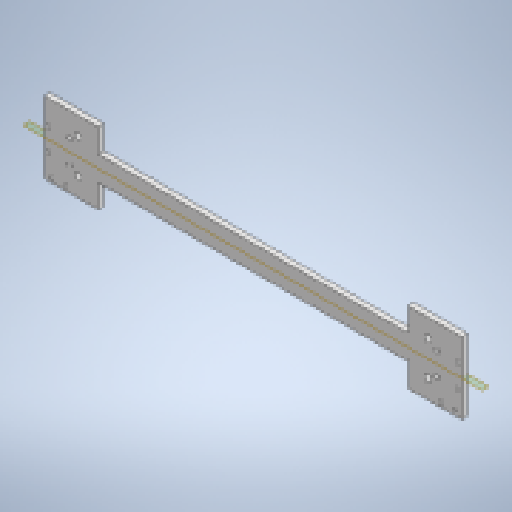
# Autodesk Inventor part: центр_рейка
Saved by Autodesk Inventor 2023.1 (Build 271208000, 208)
## iProperties
Created: 2025-12-22
Part Number: центр_рейка
Material: Типовые
Document SubType Name: Modeling
Designer: DELL
Density: 1 g/cm^3
Appearance: По умолчанию
Author: DELL
Autodesk Inventor part; units mm, degrees
ref_plane "YZ Plane" through (0, 0, 0) normal (1, 0, 0) x (0, 1, 0)
ref_plane "XZ Plane" through (0, 0, 0) normal (0, 1, 0) x (-1, 0, 0)
ref_plane "XY Plane" through (0, 0, 0) normal (0, 0, 1) x (1, 0, 0)
sketch "Эскиз1" plane through (0, 0, 0) normal (0, 0, 1) x (1, 0, 0)
  circle A0 centre (-7.5, -22.95) radius 1.5 projected
  circle A1 centre (7.5, -22.95) radius 1.5 projected
  circle A2 centre (7.5, -6.95) radius 1.5 projected
  circle A3 centre (-7.5, -6.95) radius 1.5 projected
  line L0 (-281.4, 10.05) -> (10, 10.05)
  line L1 (10, 10.05) -> (10, -39.95)
  line L2 (10, -39.95) -> (-281.4, -39.95)
  line L3 (-281.4, -39.95) -> (-281.4, 10.05)
  line L4 (-281.4, 10.05) -> (10, -39.95) construction
  line L5 (10, 10.05) -> (-281.4, -39.95) construction
  line L6 (-135.7, -14.95) -> (-135.7, -39.95) construction
  circle A4 centre (-263.9, -22.95) radius 1.5
  circle A5 centre (-278.9, -22.95) radius 1.5
  circle A6 centre (-278.9, -6.95) radius 1.5
  circle A7 centre (-263.9, -6.95) radius 1.5
  point P0 (0, 0)
  dimension "d5" = 291.4
  dimension "d8" = 2.5
  dimension "d9" = 17
  dimension "d10" = 17
  constraints: 14 end point, 4 centre point, 4 symmetric about line, 3 midpoint, 2 parallel, 1 horizontal, 1 perpendicular, 4 other
  measures "d5" distance of L1.end L2.end
  measures "d8" distance from line of L1 A2.centre
  measures "d9" distance from line of L0 A2.centre
  measures "d10" distance from line of L2 A0.centre
extrude "Выдавливание1" add sketch "Эскиз1" along normal blind 4
sketch "Эскиз3" plane through (0, 0, 4) normal (0, 0, 1) x (1, 0, 0)
  line L0 (-281.4, -39.95) -> (10, -39.95) construction
  line L1 (10, 10.05) -> (-281.4, 10.05) construction
  circle A0 centre (-257.7118, -2.95) radius 2.6
  circle A1 centre (-257.5855, -26.9497) radius 2.6
  line L2 (10, -39.95) -> (-281.4, -39.95) construction
  line L3 (-281.4, 10.05) -> (10, 10.05) construction
  line L4 (-135.7, -39.95) -> (-135.7, 10.05) construction
  circle A2 centre (-13.6882, -2.95) radius 2.6
  circle A3 centre (-13.8145, -26.9497) radius 2.6
  point P0 (0, 0)
  constraints: 6 end point, 4 centre point, 2 midpoint, 2 symmetric about line, 2 other
extrude "Выдавливание2" cut sketch "Эскиз3" against normal blind 4
sketch "Эскиз4" plane through (0, 0, 0) normal (0, 0, -1) x (-1, 0, 0)
  line L0 (27.7, 26.4968) -> (243.7, 26.4968)
  line L1 (243.7, 26.4968) -> (243.7, -6.3968)
  line L2 (243.7, -6.3968) -> (27.7, -6.3968)
  line L3 (27.7, -6.3968) -> (27.7, 26.4968)
  line L4 (-10, 10.05) -> (281.4, 10.05) projected
  line L5 (27.7, 26.4968) -> (243.7, -6.3968) construction
  line L6 (243.7, 26.4968) -> (27.7, -6.3968) construction
  point P0 (0, 0)
  point P1 (135.7, 10.05)
  point P2 (243.7, 10.05)
  dimension "d13" = 16.4468
  dimension "d14" = 216
  constraints: 12 end point, 4 midpoint, 2 parallel, 1 horizontal, 1 perpendicular
  measures "d13" distance of L1.end point (243.7, 10.05)
  measures "d14" distance of L1.end L2.end
extrude "Выдавливание3" cut sketch "Эскиз4" against normal blind 4
ref_plane "РабПлоскость1" through (-281.4, -14.95, 0) normal (0, -1, 0) x (1, 0, 0)
mirror "Зеркальное отражение1" about plane through (-281.4, -14.95, 0) normal (0, -1, 0) of "Выдавливание3"
sketch "Эскиз5" plane through (0, 0, 4) normal (0, 0, 1) x (1, 0, 0)
  circle A0 centre (4.7234, -36.95) radius 1.25 projected
  circle A1 centre (-4.7766, -36.95) radius 1.25 projected
  line L0 (-243.7, -23.5032) -> (-27.7, -23.5032) projected
  line L1 (-135.7, -23.5032) -> (-135.7, -6.3968)
  line L2 (-243.7, -6.3968) -> (-27.7, -6.3968) projected
  circle A2 centre (-276.1234, -36.95) radius 1.25
  circle A3 centre (-266.6234, -36.95) radius 1.25
  point P0 (0, 0)
  constraints: 2 centre point, 2 end point, 2 midpoint, 2 symmetric about line, 2 other
extrude "Выдавливание4" cut sketch "Эскиз5" against normal blind 10
sketch "Эскиз7" plane through (0, 0, 4) normal (0, 0, 1) x (1, 0, 0)
  circle A0 centre (-12.1342, -14.9498) radius 1.6
  circle A1 centre (-57.8342, -14.9498) radius 1.6
  point P0 (0, 0)
  constraints: 2 centre point
extrude "Выдавливание6" cut sketch "Эскиз7" against normal blind 10
